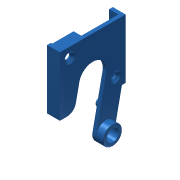
# Autodesk Inventor part: LIVER CAP
Saved by Autodesk Inventor 2014 (Build 180170000, 170)
## iProperties
Created: 2014-12-18
Part Number: LIVER CAP
Material: Steel, Cast
Document SubType Name: Modeling
Designer: Ebrahim
Density: 7.85 g/cm^3
Appearance: Cyan
Mass: 203.259 g
Surface Area: 150.482 cm^2
Volume: 25.8929 cm^3
Author: Ebrahim
Autodesk Inventor part; units mm, degrees
ref_plane "YZ Plane" through (0, 0, 0) normal (1, 0, 0) x (0, 1, 0)
ref_plane "XZ Plane" through (0, 0, 0) normal (0, 1, 0) x (-1, 0, 0)
ref_plane "XY Plane" through (0, 0, 0) normal (0, 0, 1) x (1, 0, 0)
sketch "Sketch1" plane through (0, 0, 0) normal (0, 1, 0) x (-1, 0, 0)
  line L0 (-36, 42) -> (36, 42)
  line L1 (36, 42) -> (36, -23)
  line L2 (36, -23) -> (-36, -23)
  line L3 (-36, -23) -> (-36, 42)
  line L4 (0, -36) -> (0, 55) construction
  point P0 (0, 0)
  point P1 (0, 42)
  dimension "d0" = 72
  dimension "d1" = 65
  dimension "d2" = 42
  constraints: 8 end point, 2 parallel, 1 horizontal, 1 midpoint, 1 perpendicular, 1 point on line
  measures "d0" distance of L0.start L0.end
  measures "d1" distance of L0.end L1.end
  measures "d2" distance from line of point (0, 0) L0
extrude "Extrusion1" add sketch "Sketch1" along normal blind 4
sketch "Sketch2" plane through (0, 4, 0) normal (0, 1, 0) x (1, 0, 0)
  line L0 (-36, -42) -> (36, -42) projected
  line L1 (36, -42) -> (36, 23) projected
  line L2 (36, 23) -> (-36, 23) projected
  line L3 (-36, 23) -> (-36, -42) projected
  line L4 (32, -42) -> (32, 23)
  line L5 (-32, 23) -> (-32, -42)
  line L6 (-32, -41.5) -> (-8, -41.5)
  line L7 (-8, -41.5) -> (-8, -37)
  line L8 (32, -6) -> (20, -6)
  line L9 (20, -6) -> (20, -2)
  line L10 (20, -2) -> (32, -2)
  line L11 (-32, -41.5) -> (-8, -41.5)
  line L12 (-8, -41.5) -> (-8, -37)
  line L13 (-8, -37) -> (-32, -37)
  line L14 (-32, -37) -> (-32, -41.5)
  point P0 (0, 0)
  dimension "d5" = 4
  dimension "d6" = 24
  dimension "d8" = 0.5
  dimension "d9" = 12
  dimension "d10" = 4
  dimension "d11" = 25
  constraints: 22 end point, 7 point on line, 5 perpendicular, 2 parallel, 1 horizontal
  measures "d5" distance between parallel lines of L3 L5
  measures "d6" distance of point (-32, -37) L7.end
  measures "d8" distance between parallel lines of L6 L0
  measures "d9" distance of L8.start L8.end
  measures "d10" distance of L8.end L9.end
  measures "d11" distance between parallel lines of L10 L2
extrude "Extrusion2" add sketch "Sketch2" along normal blind 10 contours L3 L2 L5 L0 | L4 L2 L1 L0 | L8 L9 L10 L4
extrude "Extrusion3" add sketch "Sketch2" along normal blind 9 contours L5 L13 L7 L6
sketch "Sketch3" plane through (0, 4, 0) normal (0, 1, 0) x (1, 0, 0)
  line L0 (-32, -42) -> (32, -42)
  line L1 (32, 23) -> (-32, 23)
  line L2 (32, 23) -> (24.280239, 60.13698)
  line L3 (10.551083, 23) -> (3.719761, 55.86302)
  line L4 (10.349326, 75.562074) -> (14.935382, 53.500217) construction
  arc A0 (24.280239, 60.13698) -> (3.719761, 55.86302) centre (14, 58) ccw
  line L5 (36, -42) -> (36, 23) construction
  line L6 (32, 23) -> (10.551083, 23)
  point P0 (0, 0)
  dimension "d16" = 21
  dimension "d17" = 22
  dimension "d18" = 100
  constraints: 8 end point, 2 parallel, 2 point on circle, 2 point on line, 2 tangent, 1 centre point, 1 collinear
  measures "d16" distance between parallel lines of L3 L2
  measures "d17" distance from line of A0.centre L5
  measures "d18" distance from line of A0.centre L0
extrude "Extrusion4" add sketch "Sketch3" against normal blind 4
hole "Hole1" at (0, 4, 0) direction (0, -1, 0) diameter 30 end through all
sketch "Sketch4" plane through (0, 4, 0) normal (0, 1, 0) x (1, 0, 0)
  circle A0 centre (0, 0) radius 15
  line L0 (3.719761, 55.86302) -> (10.551083, 23)
  line L1 (0, 0) -> (-9.827492, 47.276511) construction
  line L2 (14.697077, 3.05512) -> (4.869585, 50.33163)
  line L3 (-24.524568, 44.221391) -> (-14.697077, -3.05512)
  arc A1 (-14.697077, -3.05512) -> (14.697077, 3.05512) centre (0, 0) ccw
  arc A2 (4.869585, 50.33163) -> (-24.524568, 44.221391) centre (-9.827492, 47.276511) ccw
  point P0 (-4.913746, 23.638255)
  dimension "d28" = 15.01126
  constraints: 8 end point, 4 point on circle, 4 tangent, 2 centre point, 2 parallel, 1 collinear, 1 midpoint
  measures "d28" radius of A1
extrude "Extrusion5" cut sketch "Sketch4" against normal through all
fillet "Fillet1" radius 10 1 edges at (-20.1132, 2, -23)
sketch "Sketch5" plane through (0, 0, 0) normal (0, -1, 0) x (1, 0, 0)
  arc A0 (3.719761, -55.86302) -> (24.280239, -60.13698) centre (14, -58) ccw
  circle A1 centre (14, -58) radius 10.5
  constraints: 1 centre point, 1 coincident
extrude "Extrusion6" add sketch "Sketch5" along normal blind 8
fillet "Fillet2" radius 1 2 edges at (15.0741, 0, -47.5551) (24.4449, 0, -59.0741)
fillet "Fillet3" radius 1 1 edges at (3.5, -8, -58)
hole "Hole2" at (14, -8, -58) direction (0, 1, 0) diameter 13 end through all
sketch "Sketch6" plane through (0, 4, 0) normal (0, 1, 0) x (1, 0, 0)
  circle A0 centre (14, 58) radius 6.5
  arc A1 (24.280239, 60.13698) -> (3.719761, 55.86302) centre (14, 58) ccw
  line L0 (-14.697077, -3.05512) -> (-18.457563, 15.035219)
  circle A2 centre (18.22308, 37.684289) radius 4
  line L1 (14, 58) -> (20.5, 26.730849)
  dimension "d45" = 8
  dimension "d46" = 20.75
  constraints: 2 end point, 1 centre point, 1 parallel, 1 point on line
  measures "d45" diameter of A2
  measures "d46" distance of A2.centre A0.centre
extrude "Extrusion7" add sketch "Sketch6" along normal blind 8 contours A2 L1 | L1 A2
fillet "Fillet4" radius 1 1 edges at (14.2231, 4, -37.6843)
chamfer "Chamfer1" distance 1 angle 45 1 edges at (14.2231, 12, -37.6843)
hole "Hole3" at (-25, 0, 31) direction (0, 1, 0) diameter 6 end through all countersink diameter 12 countersink angle 90
hole "Hole4" at (25, 0, -12) direction (0, 1, 0) diameter 6 end through all countersink diameter 12 countersink angle 90
body "Solid1"
